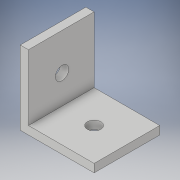
# Autodesk Inventor part: spring extentsion
Saved by Autodesk Inventor 2019 (Build 230136000, 136)
## iProperties
Created: 2019-01-19
Part Number: spring extentsion
Material: Generic
Document SubType Name: Modeling
Designer: Tiberus
Density: 1 g/cm^3
Appearance: Default
Author: Tiberus
Autodesk Inventor part; units mm, degrees
ref_plane "YZ Plane" through (0, 0, 0) normal (1, 0, 0) x (0, 1, 0)
ref_plane "XZ Plane" through (0, 0, 0) normal (0, 1, 0) x (-1, 0, 0)
ref_plane "XY Plane" through (0, 0, 0) normal (0, 0, 1) x (1, 0, 0)
sketch "Sketch1" plane through (0, 0, 0) normal (0, 1, 0) x (-1, 0, 0)
  line L0 (0, 0) -> (25.4, 0)
  line L1 (25.4, 0) -> (25.4, -25.4)
  line L2 (25.4, -25.4) -> (0, -25.4)
  line L3 (0, -25.4) -> (0, 0)
  dimension "d0" = 25.4
  dimension "d1" = 25.4
  constraints: 8 end point, 2 parallel, 1 horizontal, 1 perpendicular
  measures "d0" distance of L1.end L2.end
  measures "d1" distance of L0.end L1.end
extrude "Extrusion1" add sketch "Sketch1" along normal blind 3.175
sketch "Sketch2" plane through (0, 0, 0) normal (0, 1, 0) x (1, 0, 0)
  line L0 (-25.4, 0) -> (0, 0) construction
  line L1 (-12.7, 0) -> (-12.7, 12.7) construction
  line L2 (0, 25.4) -> (-25.4, 25.4) construction
  line L3 (-12.7, 25.4) -> (-12.7, 12.7) construction
  line L4 (-25.4, 25.4) -> (-25.4, 0) construction
  line L5 (-25.4, 12.7) -> (0, 12.7) construction
  line L6 (-25.4, 25.4) -> (-28.575, 25.4)
  line L7 (-28.575, 25.4) -> (-28.575, 0)
  line L8 (-28.575, 0) -> (-25.4, 0)
  line L9 (-25.4, 0) -> (-25.4, 25.4)
  dimension "d4" = 12.7
  dimension "d5" = 12.7
  dimension "d6" = 3.175
  constraints: 14 end point, 3 midpoint, 2 horizontal, 2 parallel, 2 vertical, 1 perpendicular
  measures "d4" distance of L1.start L1.end
  measures "d5" distance of L3.start L3.end
  measures "d6" distance of L8.end L7.end
extrude "Extrusion2" add sketch "Sketch2" along normal blind 28.575
sketch "Sketch3" plane through (0, 3.175, 0) normal (0, 1, 0) x (1, 0, 0)
  line L0 (0, 0) -> (0, 25.4) construction
  line L1 (0, 12.7) -> (-16.1864, 12.7) construction
  line L2 (0, 25.4) -> (-25.4, 25.4) construction
  line L3 (-12.7, 25.4) -> (-12.7, 5.173) construction
  circle A0 centre (-12.7, 12.7) radius 2.5797
  dimension "d9" = 5.1594
  constraints: 4 end point, 2 midpoint, 2 point on line, 1 centre point, 1 horizontal, 1 vertical
  measures "d9" diameter of A0
sketch "Sketch4" plane through (-25.4, 3.175, -25.4) normal (1, 0, 0) x (0, 0, -1)
  line L0 (0, 25.4) -> (-25.4, 25.4) construction
  line L1 (-12.7, 25.4) -> (-12.7, 8.5615) construction
  line L2 (-25.4, -3.175) -> (-25.4, 25.4) construction
  line L3 (-25.4, 11.1125) -> (0.5761, 11.1125) construction
  circle A0 centre (-12.412, 11.1125) radius 2.5797
  dimension "d10" = 5.1594
  constraints: 4 end point, 3 midpoint, 1 centre point, 1 horizontal, 1 vertical
  measures "d10" diameter of A0
extrude "Extrusion3" cut sketch "Sketch4" against normal blind 28.575
extrude "Extrusion4" cut sketch "Sketch3" against normal blind 28.575
body "Solid1"
